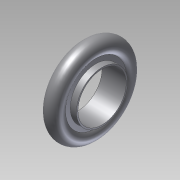
# Autodesk Inventor part: 間隔O形環
Saved by Autodesk Inventor 2016 SP1 (Build 200210100, 210)
## iProperties
Created: 2014-05-14
Part Number: 間隔O形環
Material: 一般
Document SubType Name: Modeling
Designer: Alex
Density: 1 g/cm^3
Mass: 2.06285 g
Surface Area: 18.3263 cm^2
Volume: 2.06285 cm^3
Appearance: 預設
Author: Alex
Autodesk Inventor part; units mm, degrees
ref_plane "YZ Plane" through (0, 0, 0) normal (1, 0, 0) x (0, 1, 0)
ref_plane "XZ Plane" through (0, 0, 0) normal (0, 1, 0) x (-1, 0, 0)
ref_plane "XY Plane" through (0, 0, 0) normal (0, 0, 1) x (1, 0, 0)
sketch "草圖1" plane through (0, 0, 0) normal (0, 0, 1) x (1, 0, 0)
  line L0 (0, 0) -> (81.1128, 0)
  line L1 (4.2547, -8) -> (-3.7453, -8)
  line L2 (-3.7453, -8) -> (-3.7453, -8.5)
  line L3 (-3.7453, -8.5) -> (4.2547, -8.5)
  line L4 (4.2547, -8.5) -> (4.2547, -8)
  line L5 (2.2047, -8.5) -> (-1.6953, -8.5)
  line L6 (-1.6953, -8.5) -> (-1.6953, -11.5)
  line L7 (-1.6953, -11.5) -> (2.2047, -11.5)
  line L8 (2.2047, -11.5) -> (2.2047, -8.5)
  circle A0 centre (0.2547, -11.85) radius 2.65
  point P0 (0.2547, -14.5)
  dimension "d8" = 5.3
  dimension "d0" = 8
  dimension "d1" = 3.9
  dimension "d2" = 2.05
  dimension "d3" = 1.95
  dimension "d4" = 16
  dimension "d5" = 17
  dimension "d6" = 3
  dimension "d10" = 29
  constraints: 18 end point, 4 parallel, 3 horizontal, 2 perpendicular, 1 point on line, 1 vertical alignment, 2 other
  measures "d0" distance between parallel lines of L2 L4
  measures "d1" distance between parallel lines of L8 L6
  measures "d2" distance between parallel lines of L2 L6
  measures "d3" distance from line of L6 point (0.255, -11.85)
  measures "d4" diameter of L1 L0
  measures "d5" diameter of L3 L0
  measures "d6" distance between parallel lines of L3 L7
  measures "d10" diameter of point (0.255, -14.5) L0
revolve "迴轉1" add sketch "草圖1" angle 360 about axis through (0, 0, 0) along (1, 0, 0)
equation "\"d2\" = -0.5 * d1 + 0.5 * d0"
